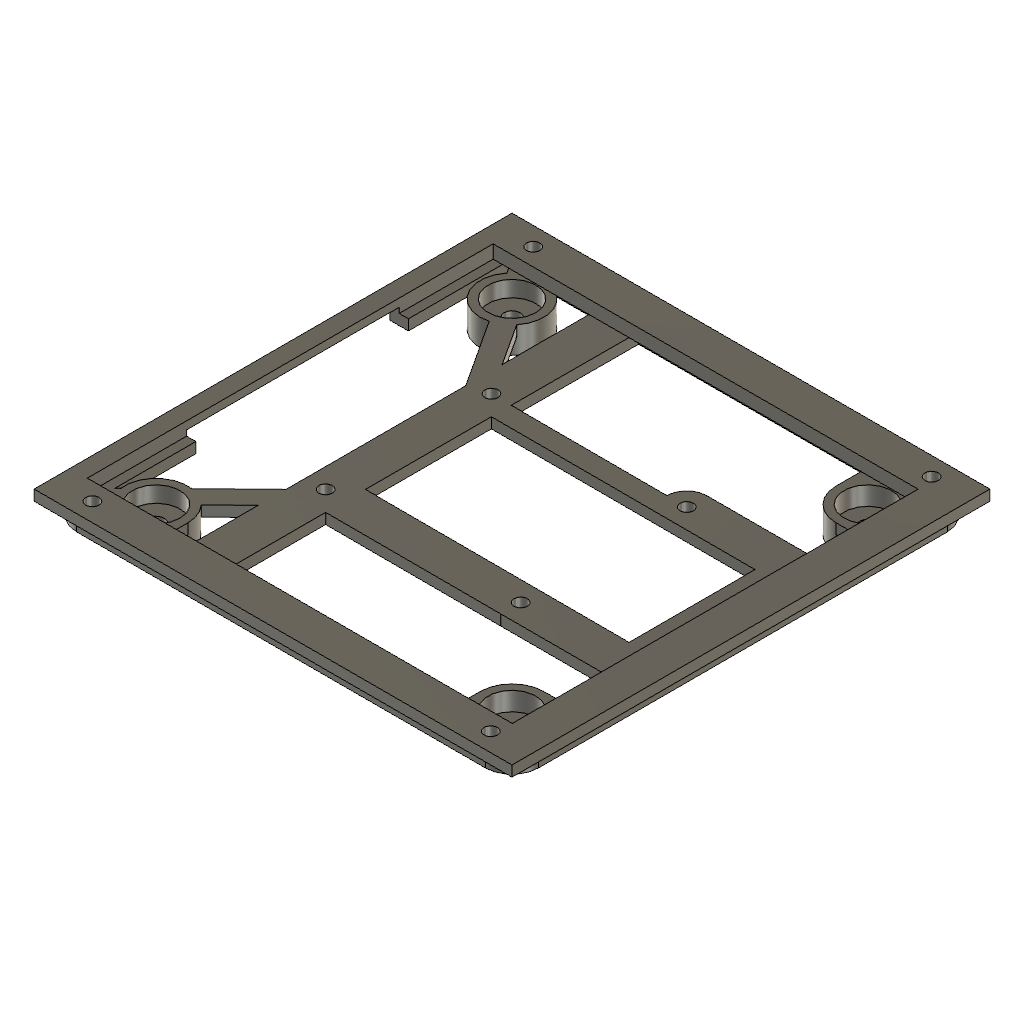
Screen Backplate (Autodesk Fusion 360 design; units mm, degrees)
Autodesk Fusion 360 part; units mm, degrees
sketch "Sketch1" plane through (0, 0, 0) normal (0, 0, 1) x (1, 0, 0)
  line L0 (0, 0) -> (90, 0)
  line L1 (90, 0) -> (90, 90)
  line L2 (90, 90) -> (0, 90)
  line L3 (0, 90) -> (0, 0)
  line L4 (0, 0) -> (5, 0)
  line L5 (5, 0) -> (5, 5)
  line L6 (5, 5) -> (0, 5)
  line L7 (0, 5) -> (0, 0)
  line L8 (90, 90) -> (85, 90)
  line L9 (85, 90) -> (85, 85)
  line L10 (85, 85) -> (90, 85)
  line L11 (90, 85) -> (90, 90)
  line L12 (85, 85) -> (5, 85)
  line L13 (5, 85) -> (5, 5)
  line L14 (5, 5) -> (85, 5)
  line L15 (85, 5) -> (85, 85)
  line L16 (90, 90) -> (87.5, 90)
  line L17 (87.5, 90) -> (87.5, 86.5)
  line L18 (87.5, 86.5) -> (90, 86.5)
  line L19 (90, 86.5) -> (90, 90)
  line L20 (87.5, 86.5) -> (82.5, 86.5)
  circle A0 centre (82.5, 86.5) radius 1.25
  line L21 (0, 0) -> (2.5, 0)
  line L22 (2.5, 0) -> (2.5, 3.5)
  line L23 (2.5, 3.5) -> (0, 3.5)
  line L24 (0, 3.5) -> (0, 0)
  line L25 (2.5, 3.5) -> (7.5, 3.5)
  line L26 (7.5, 3.5) -> (82.5, 3.5)
  line L27 (82.5, 86.5) -> (7.5, 86.5)
  circle A1 centre (7.5, 86.5) radius 1.25
  circle A2 centre (7.5, 3.5) radius 1.25
  circle A3 centre (82.5, 3.5) radius 1.25
  dimension "d1" = 90
  dimension "d2" = 90
  dimension "d3" = 5
  dimension "d4" = 5
  dimension "d5" = 5
  dimension "d6" = 5
  dimension "d7" = 2.5
  dimension "d8" = 3.5
  dimension "d10" = 5
  dimension "d12" = 2.5
  dimension "d15" = 2.5
  dimension "d16" = 3.5
  dimension "d17" = 5
  dimension "d19" = 75
  dimension "d22" = 75
  dimension "d23" = 2.5
  dimension "d26" = 2.5
  dimension "d27" = 2.5
  constraint horizontal L0
  constraint vertical L1
  constraint horizontal L2
  constraint vertical L3
  constraint coincident L0.start L3.end
  constraint horizontal L4
  constraint vertical L5
  constraint horizontal L6
  constraint vertical L7
  constraint horizontal L8
  constraint vertical L9
  constraint horizontal L10
  constraint vertical L11
  constraint horizontal L12
  constraint vertical L13
  constraint horizontal L14
  constraint vertical L15
  constraint horizontal L16
  constraint vertical L17
  constraint horizontal L18
  constraint vertical L19
  constraint perpendicular L9 L20
  constraint coincident L20.end A0.centre
  constraint horizontal L21
  constraint vertical L22
  constraint horizontal L23
  constraint vertical L24
  constraint perpendicular L22 L25
  constraint parallel L25 L26
  constraint parallel L20 L27
  constraint coincident L27.end A1.centre
  constraint coincident L25.end L26.start
  constraint coincident L26.end A3.centre
  measures "d1" distance of L0.start L0.end
  measures "d2" distance of L0.start L2.end
  measures "d3" distance of L0.start L4.end
  measures "d4" distance of L0.start L6.end
  measures "d5" distance of L1.end L8.end
  measures "d6" distance of L1.end L10.end
  measures "d7" distance of L1.end L16.end
  measures "d8" distance of L1.end L18.end
  measures "d10" distance of L17.end L20.end
  measures "d12" diameter of A0
  measures "d15" distance of L0.start L21.end
  measures "d16" distance of L0.start L23.end
  measures "d17" distance of L22.end L25.end
  measures "d19" distance of L25.end L26.end
  measures "d22" distance of L20.end L27.end
  measures "d23" diameter of A1
  measures "d26" diameter of A2
  measures "d27" diameter of A3
extrude "Extrude1" add sketch "Sketch1" along normal blind 1.5 contours L0 L3 L4 L7 L21 L22 L23 L24 | L0 L4 L5 L22 L25 | L3 L5 L6 L7 L23 L25 | L0 L1 L5 L10 L14 L15 | L2 L3 L6 L9 L12 L13 | L1 L9 L10 L11 L18 L20 | L2 L8 L9 L17 L20 | L1 L2 L8 L11 L16 L17 L18 L19 makes body 1
sketch "Sketch2" plane through (0, 0, 0) normal (0, 0, -1) x (1, 0, 0)
  circle A0 centre (7.5, -86.5) radius 1.25
  circle A1 centre (82.5, -86.5) radius 1.25
  circle A2 centre (82.5, -3.5) radius 1.25
  circle A3 centre (7.5, -3.5) radius 1.25
  line L0 (85, -5) -> (85, -85)
  line L1 (85, -85) -> (5, -85)
  line L2 (5, -85) -> (5, -5)
  line L3 (5, -5) -> (85, -5)
  line L4 (0, 0) -> (0, -90)
  line L5 (0, -90) -> (90, -90)
  line L6 (90, -90) -> (90, 0)
  line L7 (90, 0) -> (0, 0)
  line L8 (90, 0) -> (88.5, 0)
  line L9 (88.5, 0) -> (88.5, -1.5)
  line L10 (88.5, -1.5) -> (90, -1.5)
  line L11 (90, -1.5) -> (90, 0)
  line L12 (0, -90) -> (1.5, -90)
  line L13 (1.5, -90) -> (1.5, -88.5)
  line L14 (1.5, -88.5) -> (0, -88.5)
  line L15 (0, -88.5) -> (0, -90)
  line L16 (1.5, -88.5) -> (88.5, -88.5)
  line L17 (88.5, -88.5) -> (88.5, -1.5)
  line L18 (88.5, -1.5) -> (1.5, -1.5)
  line L19 (1.5, -1.5) -> (1.5, -88.5)
  dimension "d29" = 1.5
  dimension "d30" = 1.5
  dimension "d31" = 1.5
  dimension "d32" = 1.5
  constraint horizontal L8
  constraint vertical L9
  constraint horizontal L10
  constraint vertical L11
  constraint coincident L6.end L7.start
  constraint horizontal L12
  constraint vertical L13
  constraint horizontal L14
  constraint vertical L15
  constraint coincident L4.end L5.start
  constraint horizontal L16
  constraint vertical L17
  constraint horizontal L18
  constraint vertical L19
  measures "d29" distance of L6.end L8.end
  measures "d30" distance of L6.end L10.end
  measures "d31" distance of L4.end L12.end
  measures "d32" distance of L4.end L14.end
extrude "Extrude2" add sketch "Sketch2" along normal blind 2.5 contours L16 L17 L18 L19 bodies 1
sketch "Sketch3" plane through (0, 0, -2.5) normal (0, 0, -1) x (1, 0, 0)
  line L0 (5, -85) -> (5, -5)
  line L1 (5, -5) -> (85, -5)
  line L2 (85, -5) -> (85, -85)
  line L3 (85, -85) -> (5, -85)
  line L4 (88.5, -1.5) -> (1.5, -1.5)
  line L5 (1.5, -1.5) -> (1.5, -88.5)
  line L6 (1.5, -88.5) -> (88.5, -88.5)
  line L7 (88.5, -88.5) -> (88.5, -1.5)
  line L8 (88.5, -88.5) -> (1.5, -88.5)
  line L9 (1.5, -88.5) -> (1.5, -1.5)
  line L10 (1.5, -1.5) -> (88.5, -1.5)
  line L11 (88.5, -1.5) -> (88.5, -88.5)
  circle A0 centre (7.5, -86.5) radius 1.25
  circle A1 centre (82.5, -86.5) radius 1.25
  circle A2 centre (82.5, -3.5) radius 1.25
  circle A3 centre (7.5, -3.5) radius 1.25
  constraint horizontal L8
  constraint vertical L9
  constraint horizontal L10
  constraint vertical L11
  constraint coincident L4.end L5.start
  constraint coincident L6.end L7.start
extrude "Extrude3" add sketch "Sketch3" against normal blind 2 separate body contours L0 L1 L2 L3 makes body 2
sketch "Sketch4" plane through (0, 0, -0.5) normal (0, 0, 1) x (1, 0, 0)
  line L0 (85, 5) -> (85, 85)
  line L1 (5, 5) -> (85, 5)
  line L2 (5, 85) -> (5, 5)
  line L3 (85, 85) -> (5, 85)
  line L4 (5, 85) -> (5, 45.5)
  line L5 (25, 45.5) -> (25.0334, 61.1)
  line L6 (25, 45.5) -> (25.0196, 29.9)
  line L7 (25.0334, 61.1) -> (61.8833, 61.021)
  line L8 (61.8833, 61.021) -> (61.8165, 29.8211)
  circle A0 centre (61.8165, 29.8211) radius 1.25
  circle A1 centre (25.0196, 29.9) radius 1.25
  circle A2 centre (25.0334, 61.1) radius 1.25
  circle A3 centre (61.8833, 61.021) radius 1.25
  line L9 (5, 65.5) -> (5, 45.5)
  line L10 (5, 25.5) -> (5, 45.5)
  line L11 (5, 65.5) -> (-1, 65.5)
  line L12 (-1, 65.5) -> (-1, 25.5)
  line L13 (-1, 25.5) -> (5, 25.5)
  line L14 (5, 25.5) -> (5, 65.5)
  circle A4 centre (61.8165, 29.8211) radius 3.75
  circle A5 centre (25.0196, 29.9) radius 3.75
  circle A6 centre (61.8833, 61.021) radius 3.75
  circle A7 centre (25.0334, 61.1) radius 3.75
  line L15 (61.8753, 57.271) -> (85, 57.2215)
  line L16 (61.8833, 64.771) -> (85, 64.771)
  line L17 (61.8165, 26.0711) -> (85, 26.0711)
  line L18 (61.8245, 33.5711) -> (85, 33.5215)
  line L19 (28.7696, 29.9) -> (28.7696, 5)
  line L20 (21.2696, 29.9) -> (21.2696, 5)
  line L21 (21.2834, 61.1) -> (21.2834, 85)
  line L22 (28.7834, 61.0919) -> (28.8346, 85)
  line L23 (61.8753, 57.271) -> (25.0254, 57.35)
  line L24 (25.0149, 33.65) -> (61.8245, 33.5711)
  line L25 (61.8165, 26.0711) -> (25.0115, 26.15)
  line L26 (21.2696, 29.9) -> (21.2834, 61.1)
  line L27 (28.7696, 29.9) -> (28.7834, 61.0919)
  line L28 (5, 85) -> (21.8907, 59.0541)
  line L29 (25.0334, 61.1) -> (9.4746, 85)
  line L30 (5, 5) -> (27.6461, 27.2235)
  line L31 (25.0196, 29.9) -> (5, 10.254)
  line L32 (25, 45.5) -> (5, 45.5)
  dimension "d37" = 39.5
  dimension "d39" = 15.6
  dimension "d40" = 15.6
  dimension "d41" = 36.85
  dimension "d42" = 31.2
  dimension "d43" = 2.5
  dimension "d44" = 2.5
  dimension "d45" = 2.5
  dimension "d46" = 2.5
  dimension "d53" = 20
  dimension "d54" = 6
  dimension "d61" = 7.5
  dimension "d62" = 7.5
  dimension "d63" = 7.5
  dimension "d64" = 7.5
  dimension "d218" = 20
  dimension "d219" = 40
  constraint coincident L2.start L3.end
  constraint perpendicular L3 L4
  constraint perpendicular L5 L7
  constraint perpendicular L7 L8
  constraint coincident L8.end A0.centre
  constraint coincident L6.end A1.centre
  constraint coincident L5.end L7.start
  constraint coincident L7.end L8.start
  constraint vertical L9
  constraint vertical L10
  constraint horizontal L11
  constraint vertical L12
  constraint horizontal L13
  constraint vertical L14
  constraint concentric A0 A4
  constraint concentric A1 A5
  constraint concentric A3 A6
  constraint concentric A2 A7
  constraint coincident A6 L15.start
  constraint coincident L8 L15.start
  constraint coincident L0 L15.end
  constraint tangent A6 L15
  constraint coincident A6 L16.start
  constraint coincident L0 L16.end
  constraint tangent A6 L16
  constraint perpendicular L0 L16
  constraint coincident A4 L17.start
  constraint coincident L0 L17.end
  constraint tangent A4 L17
  constraint perpendicular L0 L17
  constraint coincident A4 L18.start
  constraint coincident L8 L18.start
  constraint coincident L0 L18.end
  constraint tangent A4 L18
  constraint coincident A5 L19.start
  constraint coincident L1 L19.end
  constraint tangent A5 L19
  constraint perpendicular L1 L19
  constraint coincident A5 L20.start
  constraint coincident L1 L20.end
  constraint tangent A5 L20
  constraint perpendicular L1 L20
  constraint coincident A7 L21.start
  constraint coincident L3 L21.end
  constraint tangent A7 L21
  constraint perpendicular L3 L21
  constraint coincident L7 L22.start
  constraint coincident A7 L22.start
  constraint coincident L3 L22.end
  constraint tangent A7 L22
  constraint coincident A7 L23.end
  constraint coincident L5 L23.end
  constraint coincident L6 L24.start
  constraint coincident A5 L24.start
  constraint coincident A5 L25.end
  constraint tangent A5 L25
  constraint coincident A7 L28.end
  constraint tangent A7 L28
  constraint coincident L3 L29.end
  constraint parallel L28 L29
  constraint coincident L1.start L2.end
  constraint coincident A5 L30.end
  constraint tangent A5 L30
  constraint coincident L2 L31.end
  constraint parallel L30 L31
  constraint perpendicular L14 L32
  measures "d37" distance of L2.start L4.end
  measures "d39" distance of L5.start L5.end
  measures "d40" distance of L5.start L6.end
  measures "d41" distance of L5.end L7.end
  measures "d42" distance of L7.end L8.end
  measures "d43" diameter of A0
  measures "d44" diameter of A1
  measures "d45" diameter of A2
  measures "d46" diameter of A3
  measures "d53" distance of L4.end L10.start
  measures "d54" distance of L9.start L11.end
  measures "d61" diameter of A4
  measures "d62" diameter of A5
  measures "d63" diameter of A6
  measures "d64" diameter of A7
  measures "d218" distance of L4.end L5.start
  measures "d219" distance of L9.start L10.start
extrude "Extrude4" cut sketch "Sketch4" against normal blind 2 contours L0 L1 L17 L19 L25 | L0 L8 L15 L18 | L1 L20 L30 | L8 L23 L24 L27 | L0 L3 L7 A6 A7 L16 L22 | L2 L10 L14 L20 L26 L31 L32 | L7 L8 A3 | L7 L8 A3 | L6 A1 L31 | L6 A1 L31 | L2 L4 L9 L14 L26 L28 L32 | L3 L21 L29 | L5 L7 A2 | L7 A2 L29 | L5 A2 L29 | A0 bodies 2
extrude "Extrude5" cut sketch "Sketch4" against normal blind 8 contours L2 L10 L14 L20 L26 L31 L32 | L2 L4 L9 L10 L11 L12 L13 L14 | L2 L4 L9 L14 L26 L28 L32 bodies 1 2
extrude "Extrude7" cut 1 faces at (3.8333, 52.1667, -0.5) along direction (0, 0, 1) blind 1 on bodies 1 bodies 1
sketch "Sketch28" plane through (0, 0, -0.5) normal (0, 0, 1) x (-1, 0, 0)
  line L0 (-21.2696, -26.22) -> (-5, -10.254)
  line L1 (-5, -10.254) -> (-5, -5)
  line L2 (-5, -5) -> (-21.2696, -20.966)
  line L3 (-21.2696, -20.966) -> (-21.2696, -5)
  line L4 (-21.2696, -5) -> (-28.7696, -5)
  line L5 (-28.7696, -5) -> (-28.7696, -26.142)
  line L6 (-28.7696, -26.142) -> (-61.8165, -26.0711)
  line L7 (-85, -26.0711) -> (-85, -33.5215)
  line L8 (-85, -33.5215) -> (-61.8245, -33.5711)
  line L9 (-28.7712, -33.642) -> (-28.7817, -57.3419)
  line L10 (-28.7817, -57.3419) -> (-85, -57.2215)
  line L11 (-85, -57.2215) -> (-85, -64.771)
  line L12 (-85, -64.771) -> (-61.8833, -64.771)
  arc A0 (-61.8833, -64.771) -> (-58.1333, -61.0291) centre (-61.8833, -61.021) ccw
  line L13 (-58.1333, -61.0291) -> (-28.7834, -61.0919)
  line L14 (-28.7834, -61.0919) -> (-28.8346, -85)
  line L15 (-28.8346, -85) -> (-21.2834, -85)
  line L16 (-21.2834, -85) -> (-21.2834, -66.8604)
  line L17 (-21.2834, -66.8604) -> (-9.4746, -85)
  line L18 (-9.4746, -85) -> (-5, -85)
  line L19 (-5, -85) -> (-21.2829, -59.9876)
  circle A1 centre (-25.0196, -29.9) radius 1.25
  circle A2 centre (-25.0334, -61.1) radius 1.25
  circle A3 centre (-61.8165, -29.8211) radius 1.25
  circle A4 centre (-61.8833, -61.021) radius 1.25
  line L20 (-5, -5) -> (-85, -5)
  line L21 (-85, -5) -> (-85, -6.8)
  line L22 (-85, -6.8) -> (-5, -6.8)
  line L23 (-5, -6.8) -> (-5, -5)
  line L24 (-5, -85) -> (-85, -85)
  line L25 (-85, -85) -> (-85, -83.2)
  line L26 (-85, -83.2) -> (-5, -83.2)
  line L27 (-5, -83.2) -> (-5, -85)
  line L28 (-5, -83.2) -> (-3.25, -83.2)
  line L29 (-3.25, -83.2) -> (-3.25, -6.8)
  line L30 (-3.25, -6.8) -> (-5, -6.8)
  line L31 (-5, -6.8) -> (-5, -83.2)
  line L32 (-85, -83.2) -> (-83.25, -83.2)
  line L33 (-83.25, -83.2) -> (-83.25, -6.8)
  line L34 (-83.25, -6.8) -> (-85, -6.8)
  line L35 (-85, -6.8) -> (-85, -83.2)
  line L36 (-61.8165, -26.0711) -> (-85, -26.0711)
  line L37 (-61.8245, -33.5711) -> (-28.7712, -33.642)
  line L38 (-21.2829, -59.9876) -> (-21.2696, -29.9)
  line L39 (-21.2696, -29.9) -> (-21.2696, -26.22)
  dimension "d200" = 80
  dimension "d201" = 1.8
  dimension "d202" = 1.8
  dimension "d212" = 1.75
  dimension "d213" = 1.75
  constraint horizontal L20
  constraint vertical L21
  constraint horizontal L22
  constraint vertical L23
  constraint coincident L1.end L2.start
  constraint horizontal L24
  constraint vertical L25
  constraint horizontal L26
  constraint vertical L27
  constraint coincident L18.end L19.start
  constraint horizontal L28
  constraint vertical L29
  constraint horizontal L30
  constraint vertical L31
  constraint horizontal L32
  constraint vertical L33
  constraint horizontal L34
  constraint vertical L35
  measures "d200" distance of L1.end L20.end
  measures "d201" distance of L1.end L22.end
  measures "d202" distance of L18.end L26.end
  measures "d212" distance of L26.end L28.end
  measures "d213" distance of L25.end L32.end
extrude "Extrude31" add sketch "Sketch28" along normal blind 2 contours L1 L2 L22 L23 | L19 L26 L27 | L2 L3 L20 L22 | L17 L18 L19 L24 L26 | L3 L4 L5 L20 L22 | L16 L17 L24 L26 | L5 L20 L21 L22 L34 | L14 L15 L16 L24 L26 | L14 L24 L25 L26 L32 bodies 1 2
extrude "Extrude32" cut sketch "Sketch28" along normal blind 2 contours L1 L28 L29 L30 L31 bodies 1
extrude "Extrude33" add sketch "Sketch28" along normal blind 2 contours L22 L33 L34 L35 L36 | L7 L8 L33 L35 L36 | L12 L26 L32 L33 L35 | L8 L10 L33 L35 | L10 L11 L12 L33 L35 bodies 1
sketch "Sketch24" plane through (0, 0, -2.5) normal (0, 0, -1) x (1, 0, 0)
  line L0 (5, -65.5) -> (1.5, -65.5)
  line L1 (1.5, -88.5) -> (88.5, -88.5)
  line L2 (88.5, -88.5) -> (88.5, -1.5)
  line L3 (88.5, -1.5) -> (1.5, -1.5)
  line L4 (1.5, -65.5) -> (1.5, -88.5)
  line L5 (1.5, -25.5) -> (5, -25.5)
  line L6 (5, -85) -> (5, -65.5)
  line L7 (28.7696, -5) -> (85, -5)
  line L8 (85, -33.5215) -> (85, -57.2215)
  line L9 (21.2834, -85) -> (9.4746, -85)
  line L10 (88.5, -1.5) -> (78.5, -1.5)
  line L11 (78.5, -1.5) -> (78.5, -11.5)
  line L12 (78.5, -11.5) -> (88.5, -11.5)
  line L13 (88.5, -11.5) -> (88.5, -1.5)
  line L14 (78.5, -11.5) -> (78.5, -78.5)
  circle A0 centre (78.5, -78.5) radius 1.5
  circle A1 centre (78.5, -11.5) radius 1.5
  circle A2 centre (11.5, -11.5) radius 1.5
  circle A3 centre (78.5, -11.5) radius 6
  circle A4 centre (11.5, -11.5) radius 6
  circle A5 centre (78.5, -78.5) radius 6
  line L15 (78.5, -78.5) -> (88.5, -78.5)
  line L16 (88.5, -78.5) -> (88.5, -88.5)
  line L17 (88.5, -88.5) -> (78.5, -88.5)
  line L18 (78.5, -88.5) -> (78.5, -78.5)
  line L19 (72.5, -78.5) -> (72.5, -88.5)
  line L20 (17.5, -11.5) -> (17.5, -5)
  line L21 (72.5, -11.5) -> (72.5, -1.5)
  line L22 (78.5, -17.5) -> (88.5, -17.5)
  line L23 (78.5, -72.5) -> (85, -72.5)
  line L24 (10.3167, -5.6178) -> (5, -6.6874)
  line L25 (5, -25.5) -> (5, -10.254)
  line L26 (5, -10.254) -> (21.2696, -26.22)
  line L27 (21.2696, -26.22) -> (21.2696, -29.9)
  line L28 (21.2829, -59.9876) -> (5, -85)
  line L29 (85, -57.2215) -> (28.7817, -57.3419)
  line L30 (28.7817, -57.3419) -> (28.7712, -33.642)
  line L31 (28.7712, -33.642) -> (61.8245, -33.5711)
  line L32 (9.4746, -85) -> (21.2834, -66.8604)
  line L33 (21.2834, -66.8604) -> (21.2834, -85)
  line L34 (28.8346, -85) -> (28.7834, -61.0919)
  line L35 (28.7834, -61.0919) -> (58.1333, -61.0291)
  arc A6 (58.1333, -61.0291) -> (61.8833, -64.771) centre (61.8833, -61.021) ccw
  line L36 (61.8833, -64.771) -> (85, -64.771)
  line L37 (85, -64.771) -> (85, -85)
  line L38 (85, -85) -> (28.8346, -85)
  line L39 (85, -26.0711) -> (61.8165, -26.0711)
  line L40 (28.7696, -26.142) -> (28.7696, -5)
  line L41 (85, -5) -> (85, -26.0711)
  circle A7 centre (25.0196, -29.9) radius 1.25
  circle A8 centre (25.0334, -61.1) radius 1.25
  circle A9 centre (61.8165, -29.8211) radius 1.25
  circle A10 centre (61.8833, -61.021) radius 1.25
  line L42 (21.2696, -5) -> (21.2696, -20.966)
  line L43 (21.2696, -20.966) -> (5, -5)
  line L44 (5, -5) -> (21.2696, -5)
  line L45 (1.5, -1.5) -> (1.5, -25.5)
  circle A11 centre (7.5, -3.5) radius 1.25
  circle A12 centre (82.5, -3.5) radius 1.25
  circle A13 centre (82.5, -86.5) radius 1.25
  circle A14 centre (7.5, -86.5) radius 1.25
  line L46 (78.5, -78.5) -> (11.5, -78.5)
  circle A15 centre (11.5, -78.5) radius 1.5
  circle A16 centre (11.5, -78.5) radius 6
  line L47 (21.2696, -29.9) -> (21.2829, -59.9876)
  line L48 (61.8245, -33.5711) -> (85, -33.5215)
  line L49 (61.8165, -26.0711) -> (28.7696, -26.142)
  dimension "d168" = 10
  dimension "d169" = 10
  dimension "d172" = 67
  dimension "d174" = 3
  dimension "d176" = 3
  dimension "d177" = 3
  dimension "d178" = 12
  dimension "d179" = 12
  dimension "d181" = 12
  dimension "d187" = 10
  dimension "d209" = 67
  dimension "d210" = 3
  dimension "d211" = 12
  constraint horizontal L10
  constraint vertical L11
  constraint horizontal L12
  constraint vertical L13
  constraint perpendicular L12 L14
  constraint coincident L14.end A0.centre
  constraint coincident L11.end L12.start
  constraint concentric A1 A3
  constraint concentric A0 A5
  constraint horizontal L15
  constraint vertical L16
  constraint horizontal L17
  constraint vertical L18
  constraint coincident L1.end L2.start
  constraint coincident A5 L19.start
  constraint tangent A5 L19
  constraint coincident A4 L20.start
  constraint coincident L7 L20.end
  constraint perpendicular L7 L20
  constraint coincident A3 L21.start
  constraint tangent A3 L21
  constraint coincident L14 L22.start
  constraint coincident A3 L22.start
  constraint coincident A5 L23.start
  constraint coincident L14 L23.start
  constraint coincident L8 L23.end
  constraint tangent A5 L23
  constraint coincident A4 L24.start
  constraint coincident L6 L24.end
  constraint tangent A4 L24
  constraint horizontal L46
  constraint coincident L46.end A15.centre
  constraint concentric A15 A16
  measures "d168" distance of L2.end L10.end
  measures "d169" distance of L2.end L12.end
  measures "d172" distance of L11.end L14.end
  measures "d174" diameter of A0
  measures "d176" diameter of A1
  measures "d177" diameter of A2
  measures "d178" diameter of A3
  measures "d179" diameter of A4
  measures "d181" diameter of A5
  measures "d187" distance of L22.start L22.end
  measures "d209" distance of L14.end L46.end
  measures "d210" diameter of A15
  measures "d211" diameter of A16
extrude "Extrude25" add sketch "Sketch24" against normal blind 2 contours L28 A16 | L28 L32 A16 | L1 L18 L19 L38 | L3 L5 L7 L14 A4 L21 L25 L26 L27 L28 L29 L30 L31 L32 L33 L34 L35 A6 L36 L39 L40 L42 L43 L44 L45 L46 A16 L47 L48 L49 | L32 L46 A16 | L1 L2 L15 L16 L17 L18 L37 L38 | A5 L18 L19 L38 | L32 L46 A16 | A5 L15 L18 L37 L38 | A0 A5 L18 L46 | L14 A0 A5 L46 | L2 L8 L14 L15 L22 L29 L36 L37 L39 L41 L48 | A0 A5 L15 L18 | L14 A0 A5 L15 | A5 L15 L23 L37 | L2 L12 L22 L41 | A2 A4 L26 L43 | A4 L26 | L2 L3 L7 L10 L11 L12 L13 L41 | L12 A3 L22 L41 | L8 L14 L29 L48 | A2 A4 L43 | L7 L11 L12 A3 L41 | L11 L14 A1 A3 | L12 L14 A1 A3 | A4 L24 L43 | A4 L20 L24 L43 L44 | A2 L43 | L3 L7 L11 L21 | L11 L12 A1 A3 | L7 L11 A3 L21 | A11 | A12 | A13 picked at (10.9091, -11.9541) bodies 1
extrude "Extrude27" cut sketch "Sketch24" against normal blind 2 contours A0 L18 L46 | L14 A0 L46 | A0 L15 L18 | L14 A0 L15 | A2 L43 | A2 L43 | L11 L14 A1 | L12 L14 A1 | L11 L12 A1 | A15 bodies 1
extrude "Extrude26" add sketch "Sketch24" along normal blind 3 contours L28 A16 | L28 L32 A16 | L32 L46 A16 | L32 L46 A16 | A0 A5 L18 L46 | L14 A0 A5 L46 | A0 A5 L15 L18 | L14 A0 A5 L15 | A2 A4 L26 L43 | A4 L26 | A2 A4 L43 | L11 L14 A1 A3 | L12 L14 A1 A3 | L11 L12 A1 A3 bodies 1
sketch "Sketch25" plane through (0, 0, -0.5) normal (0, 0, 1) x (-1, 0, 0)
  circle A0 centre (-78.5, -11.5) radius 1.5
  line L0 (-83.25, -17.5) -> (-78.5, -17.5)
  arc A1 (-78.5, -17.5) -> (-72.5, -11.5) centre (-78.5, -11.5) ccw
  line L1 (-72.5, -11.5) -> (-72.5, -6.8)
  circle A2 centre (-78.5, -11.5) radius 4.5
  line L2 (-72.5, -6.8) -> (-83.25, -6.8)
  line L3 (-83.25, -6.8) -> (-83.25, -17.5)
  dimension "d190" = 9
  constraint concentric A0 A2
  measures "d190" diameter of A2
extrude "Extrude28" cut sketch "Sketch25" against normal blind 3.5 contours A2 bodies 1
sketch "Sketch26" plane through (0, 0, -0.5) normal (0, 0, 1) x (-1, 0, 0)
  circle A0 centre (-11.5, -11.5) radius 1.5
  line L0 (-28.7696, -6.8) -> (-28.7696, -26.142)
  line L1 (-28.7696, -26.142) -> (-61.8165, -26.0711)
  line L2 (-78.5, -33.5354) -> (-61.8245, -33.5711)
  line L3 (-28.7712, -33.642) -> (-28.7817, -57.3419)
  line L4 (-28.7817, -57.3419) -> (-78.5, -57.2354)
  line L5 (-83.25, -64.771) -> (-61.8833, -64.771)
  arc A1 (-61.8833, -64.771) -> (-58.1333, -61.0291) centre (-61.8833, -61.021) ccw
  line L6 (-58.1333, -61.0291) -> (-28.7834, -61.0919)
  line L7 (-28.7834, -61.0919) -> (-28.8308, -83.2)
  line L8 (-6.1718, -83.2) -> (-6.8019, -82.232)
  line L9 (-21.2696, -26.22) -> (-12.3256, -17.4429)
  arc A2 (-12.3256, -17.4429) -> (-5.5426, -10.7865) centre (-11.5, -11.5) ccw
  circle A3 centre (-11.5, -78.5) radius 4.5
  circle A4 centre (-11.5, -11.5) radius 4.5
  line L10 (-21.2696, -6.8) -> (-28.7696, -6.8)
  line L11 (-21.2696, -20.966) -> (-21.2696, -6.8)
  line L12 (-28.8308, -83.2) -> (-21.2834, -83.2)
  line L13 (-5, -10.254) -> (-5, -25.5)
  line L14 (-17.5, -6.8) -> (-17.5, -11.5)
  line L15 (-15.8426, -15.6403) -> (-21.2696, -20.966)
  arc A5 (-16.1636, -74.725) -> (-15.2296, -83.2) centre (-11.5, -78.5) ccw
  circle A6 centre (-11.5, -78.5) radius 1.5
  circle A7 centre (-25.0196, -29.9) radius 1.25
  circle A8 centre (-25.0334, -61.1) radius 1.25
  circle A9 centre (-61.8165, -29.8211) radius 1.25
  circle A10 centre (-61.8833, -61.021) radius 1.25
  line L16 (-21.2834, -83.2) -> (-21.2834, -66.8604)
  line L17 (-21.2834, -66.8604) -> (-16.1636, -74.725)
  line L18 (-83.25, -26.0711) -> (-83.25, -64.771)
  line L19 (-5.5426, -10.7865) -> (-5, -10.254)
  line L20 (-5, -25.5) -> (-3.25, -25.5)
  line L21 (-3.25, -25.5) -> (-3.25, -6.8)
  line L22 (-3.25, -6.8) -> (-17.5, -6.8)
  arc A11 (-17.5, -11.5) -> (-15.8426, -15.6403) centre (-11.5, -11.5) ccw
  line L23 (-61.8165, -26.0711) -> (-83.25, -26.0711)
  line L24 (-21.2829, -59.9876) -> (-21.2696, -29.9)
  line L25 (-21.2696, -29.9) -> (-21.2696, -26.22)
  line L26 (-61.8245, -33.5711) -> (-28.7712, -33.642)
  line L27 (-78.5, -57.2354) -> (-78.5, -33.5354)
  line L28 (-15.2296, -83.2) -> (-6.1718, -83.2)
  arc A12 (-6.8019, -82.232) -> (-13.0115, -72.6935) centre (-11.5, -78.5) ccw
  line L29 (-13.0115, -72.6935) -> (-21.2829, -59.9876)
  dimension "d193" = 9
  dimension "d194" = 9
  constraint concentric A0 A4
  measures "d193" diameter of A3
  measures "d194" diameter of A4
extrude "Extrude29" cut sketch "Sketch26" against normal blind 3 contours A3 | A4 | A6 bodies 1
sketch "Sketch27" plane through (0, 0, -0.5) normal (0, 0, 1) x (-1, 0, 0)
  circle A0 centre (-78.5, -78.5) radius 1.5
  line L0 (-72.5, -83.2) -> (-72.5, -78.5)
  arc A1 (-72.5, -78.5) -> (-78.5, -72.5) centre (-78.5, -78.5) ccw
  line L1 (-78.5, -72.5) -> (-83.25, -72.5)
  circle A2 centre (-78.5, -78.5) radius 4.5
  line L2 (-83.25, -83.2) -> (-72.5, -83.2)
  line L3 (-83.25, -72.5) -> (-83.25, -83.2)
  dimension "d197" = 9
  constraint concentric A0 A2
  measures "d197" diameter of A2
extrude "Extrude30" cut sketch "Sketch27" against normal blind 3.5 contours A2 bodies 1
extrude "Extrude34" add 1 faces at (87.75, 57.7333, 1.5) along direction (0, 0, 1) blind 0.5 on bodies 1 bodies 1
fillet "Fillet16" radius 5 4 edges at (1.5, 1.5, -1.25) (88.5, 1.5, -1.25) (88.5, 88.5, -1.25) (1.5, 88.5, -1.25) on bodies 1
sketch "Sketch29" plane through (90, 0, 0) normal (1, 0, 0) x (0, 1, 0)
  line L0 (0, 0) -> (90, 0)
  line L1 (90, 0) -> (90, 2)
  line L2 (90, 2) -> (0, 2)
  line L3 (0, 2) -> (0, 0)
  line L4 (0, 0) -> (0, 4.5)
  line L5 (0, 0) -> (-4.5, 0)
  line L6 (0, 4.5) -> (-4.5, 0)
  line L7 (90, 0) -> (94.5, 0)
  line L8 (90, 0) -> (90, 4.5)
  line L9 (90, 4.5) -> (94.5, 0)
  dimension "d224" = 4.5
  dimension "d225" = 4.5
  dimension "d226" = 4.5
  dimension "d227" = 4.5
  constraint coincident L0.start L3.end
  constraint perpendicular L2 L4
  constraint perpendicular L4 L5
  constraint coincident L0.end L1.start
  constraint perpendicular L1 L7
  constraint perpendicular L7 L8
  measures "d224" distance of L0.start L4.end
  measures "d225" distance of L0.start L5.end
  measures "d226" distance of L0.end L7.end
  measures "d227" distance of L0.end L8.end
sketch "Sketch30" plane through (0, 90, 0) normal (0, 1, 0) x (-1, 0, 0)
  line L0 (-90, 0) -> (0, 0)
  line L1 (0, 0) -> (0, 2)
  line L2 (0, 2) -> (-90, 2)
  line L3 (-90, 2) -> (-90, 0)
  line L4 (-90, 0) -> (-94.5, 0)
  line L5 (-90, 0) -> (-90, 4.5)
  line L6 (0, 0) -> (4.5, 0)
  line L7 (0, 0) -> (0, 4.5)
  line L8 (-90, 4.5) -> (-94.5, 0)
  line L9 (0, 4.5) -> (4.5, 0)
  dimension "d232" = 4.5
  dimension "d233" = 4.5
  dimension "d234" = 4.5
  dimension "d235" = 4.5
  constraint coincident L0.start L3.end
  constraint perpendicular L3 L4
  constraint perpendicular L4 L5
  constraint coincident L0.end L1.start
  constraint perpendicular L1 L6
  constraint perpendicular L6 L7
  measures "d232" distance of L0.start L4.end
  measures "d233" distance of L0.start L5.end
  measures "d234" distance of L0.end L6.end
  measures "d235" distance of L0.end L7.end
extrude "Extrude35" [suppressed]
extrude "Extrude36" [suppressed]
extrude "Extrude37" [suppressed]
extrude "Extrude38" [suppressed]
extrude "Extrude39" [suppressed]
extrude "Extrude40" [suppressed]
sketch "Sketch31" plane through (0, 0, 0) normal (0, 0, -1) x (1, 0, 0)
  line L0 (6.5, -1.5) -> (83.5, -1.5)
  arc A0 (88.5, -6.5) -> (83.5, -1.5) centre (83.5, -6.5) ccw
  line L1 (88.5, -6.5) -> (88.5, -83.5)
  arc A1 (83.5, -88.5) -> (88.5, -83.5) centre (83.5, -83.5) ccw
  line L2 (83.5, -88.5) -> (6.5, -88.5)
  arc A2 (1.5, -83.5) -> (6.5, -88.5) centre (6.5, -83.5) ccw
  line L3 (1.5, -83.5) -> (1.5, -65.5)
  line L4 (1.5, -65.5) -> (1.5, -25.5)
  line L5 (1.5, -25.5) -> (1.5, -6.5)
  arc A3 (6.5, -1.5) -> (1.5, -6.5) centre (6.5, -6.5) ccw
  line L6 (-4.5, 4.5) -> (-4.5, -94.5)
  line L7 (-4.5, -94.5) -> (94.5, -94.5)
  line L8 (94.5, -94.5) -> (94.5, 4.5)
  line L9 (94.5, 4.5) -> (-4.5, 4.5)
  line L10 (-4.5, -94.5) -> (0, -94.5)
  dimension "d258" = 4.5
  constraint coincident L6.end L7.start
  constraint perpendicular L6 L10
  measures "d258" distance of L6.end L10.end
fillet "Fillet17" [suppressed]
